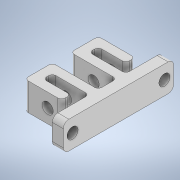
# Autodesk Inventor part: Festoon_Carriage
Saved by Autodesk Inventor 2022 (Build 260153000, 153)
## iProperties
Created: 2022-02-27
Part Number: Festoon_Carriage
Material: Generic
Document SubType Name: Modeling
Designer: Jorian Brusind
Density: 1 g/cm^3
Appearance: Default
Author: Jorian Brusind
Autodesk Inventor part; units mm, degrees
ref_plane "YZ Plane" through (0, 0, 0) normal (1, 0, 0) x (0, 1, 0)
ref_plane "XZ Plane" through (0, 0, 0) normal (0, 1, 0) x (-1, 0, 0)
ref_plane "XY Plane" through (0, 0, 0) normal (0, 0, 1) x (1, 0, 0)
sketch "Sketch1" plane through (0, 0, 0) normal (0, 1, 0) x (-1, 0, 0)
  line L0 (-3, -30) -> (3, -30)
  line L1 (3, -30) -> (3, 30)
  line L2 (3, 30) -> (-3, 30)
  line L3 (-3, 30) -> (-3, -30)
  line L4 (-3, -30) -> (3, 30) construction
  line L5 (3, -30) -> (-3, 30) construction
  line L6 (3, 30) -> (3, 20)
  line L7 (3, 20) -> (28, 20)
  line L8 (28, 20) -> (28, 5)
  line L9 (28, 5) -> (3, 5)
  line L10 (3, 5) -> (3, 20)
  line L11 (15.5, 20) -> (10.5, 20)
  line L12 (15.5, 20) -> (8, 20)
  line L13 (3, 20) -> (8, 20)
  line L14 (8, 20) -> (8, 15)
  line L15 (8, 15) -> (3, 15)
  line L16 (3, 15) -> (3, 20)
  line L17 (3, 15) -> (23, 15)
  line L18 (23, 15) -> (23, 10)
  line L19 (23, 10) -> (3, 10)
  line L20 (3, 10) -> (3, 15)
  line L21 (0, 0) -> (20, 0)
  line L22 (3, -20) -> (28, -20)
  line L23 (28, -20) -> (28, -5)
  line L24 (28, -5) -> (3, -5)
  line L25 (8, -20) -> (8, -15)
  line L26 (8, -15) -> (3, -15)
  line L27 (3, -15) -> (23, -15)
  line L28 (23, -15) -> (23, -10)
  line L29 (23, -10) -> (3, -10)
  dimension "d0" = 6
  dimension "d1" = 60
  dimension "d2" = 10
  dimension "d3" = 25
  dimension "d4" = 15
  dimension "d8" = 5
  dimension "d9" = 5
  dimension "d10" = 20
  dimension "d11" = 5
  dimension "d12" = 20
  constraints: 60 end point, 10 symmetric about line, 8 parallel, 6 horizontal, 4 perpendicular, 3 midpoint, 2 point on line
  measures "d0" distance of L2.end L1.end
  measures "d1" distance of L1.end L0.end
  measures "d2" distance of L1.end L6.end
  measures "d3" distance of L8.end L9.end
  measures "d4" distance of L7.end L8.end
  measures "d8" distance of L14.end L15.end
  measures "d9" distance of L13.end L14.end
  measures "d10" distance of L18.end L19.end
  measures "d11" distance of L17.end L18.end
  measures "d12" distance of L21.start L21.end
extrude "Extrusion1" add sketch "Sketch1" along normal blind 15 contours L3 L2 L1 L0 | L25 L27 L28 L29 L1 L24 L23 L22 | L7 L8 L9 L1 L19 L18 L17 L14
sketch "Sketch2" plane through (-28, 0, 20) normal (0, 0, 1) x (1, 0, 0)
  line L0 (20, 0) -> (20, 15) projected
  line L1 (20, 7.5) -> (12.5, 7.5)
  circle A0 centre (12.5, 7.5) radius 3
  point P0 (28, 0)
  dimension "d15" = 7.5
  dimension "d16" = 6
  constraints: 2 end point, 1 centre point, 1 coincident, 1 horizontal, 1 midpoint
  measures "d15" distance of L1.start L1.end
  measures "d16" diameter of A0
extrude "Extrusion2" cut sketch "Sketch2" against normal through all
fillet "Fillet1" radius 2 16 edges at (-8, 7.5, 20) (-8, 7.5, 15) (-3, 7.5, 10) (-28, 7.5, 20) (-28, 7.5, 5) (-23, 7.5, 10) (-23, 7.5, 15) (-23, 7.5, -15) (-23, 7.5, -10) (-28, 7.5, -5) (-28, 7.5, -20) (-8, 7.5, -20) (-8, 7.5, -15) (-3, 7.5, -10) (-3, 7.5, 5) (-3, 7.5, -5)
sketch "Sketch3" plane through (-3, 0, -30) normal (-1, 0, 0) x (0, 0, 1)
  line L0 (60, 0) -> (60, 15) projected
  line L1 (60, 7.5) -> (55, 7.5)
  line L2 (0, 0) -> (0, 15) projected
  line L3 (0, 7.5) -> (5, 7.5)
  circle A0 centre (55, 7.5) radius 3
  circle A1 centre (5, 7.5) radius 3
  point P0 (30, 0)
  dimension "d20" = 5
  dimension "d21" = 5
  dimension "d22" = 6
  dimension "d23" = 6
  constraints: 4 end point, 2 centre point, 2 coincident, 2 horizontal, 2 midpoint
  measures "d20" distance of L1.start L1.end
  measures "d21" distance of L3.start L3.end
  measures "d22" diameter of A0
  measures "d23" diameter of A1
extrude "Extrusion3" cut sketch "Sketch3" against normal through all
fillet "Fillet2" radius 3 4 edges at (0, 15, 30) (0, 15, -30) (0, 0, -30) (0, 0, 30)
body "Solid1"
